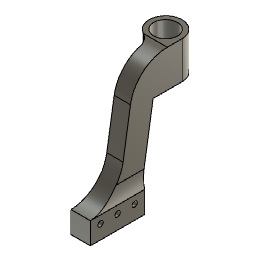
JRCNC0014 v32 (Autodesk Fusion 360 design; units mm, degrees)
Autodesk Fusion 360 part; units mm, degrees
sketch "Sketch1" plane through (0, 0, 0) normal (0, 0, 1) x (1, 0, 0)
  circle A0 centre (0, 0) radius 7.625
  circle A1 centre (0, 0) radius 10.625
  line L0 (0, 0) -> (0, -7.5) construction
  line L1 (10.625, 0) -> (-10.625, 0)
  line L2 (-10.625, 0) -> (-10.625, -15)
  line L3 (-10.625, -15) -> (10.625, -15)
  line L4 (10.625, -15) -> (10.625, 0)
  line L5 (10.625, 0) -> (-10.625, -15) construction
  line L6 (-10.625, 0) -> (10.625, -15) construction
  line L7 (0, 0) -> (0, -15)
  point P0 (0, -7.5)
  dimension "d2" = 3
  dimension "d3" = 15.25
  dimension "d10" = 15
  constraint coincident A0.centre A1.centre
  constraint vertical L0
  constraint horizontal L1
  constraint perpendicular L1 L2
  constraint parallel L1 L3
  constraint parallel L2 L4
  constraint coincident A1 L1.start
  constraint coincident L5 P0
  constraint coincident L6 P0
  constraint coincident P0 L0.end
  constraint midpoint L3 L7.end
  measures "d2" distance of A0 A1
  measures "d3" diameter of A0
  measures "d10" distance of L1.end L2.end
extrude "Extrude1" add sketch "Sketch1" along normal blind 24 contours A0 A1 L1 L7 | A0 A1 L1 | A0 A1 L1 L7 | A1 L3 L4 L7 picked at (1.863551, -9.419618) picked at (-7.385661, 6.132809) picked at (-0.865749, -9.56308) picked at (4.539469, -13.398204)
sketch "Sketch2" plane through (10.625, 0, 0) normal (1, 0, 0) x (0, -1, 0)
  line L0 (15, 0) -> (0, 0)
  line L1 (0, 0) -> (0, -24)
  line L2 (0, -24) -> (15, -24)
  line L3 (15, -24) -> (15, 0)
  line L4 (15, -24) -> (30, -24)
  line L5 (30, -24) -> (41.250246, 46)
  line L6 (41.250246, 46) -> (26.057754, 46)
  line L7 (26.057754, 46) -> (18.656827, -0.049205)
  line L8 (18.656827, -0.049205) -> (15, 0)
  point P0 (33.654, 46)
  dimension "d30" = 30
  dimension "d31" = 70
  dimension "d32" = 33.654
  dimension "d34" = 15
  constraint coincident L2.end L3.start
  constraint perpendicular L3 L4
  constraint perpendicular L3 L6
  constraint parallel L5 L7
  constraint coincident L0.start L3.end
  constraint midpoint L6 P0
  measures "d30" distance of L1 L4.end
  measures "d32" horizontal distance of L0.end P0
  measures "d34" distance of L5 L7
extrude "Extrude2" add sketch "Sketch2" against normal blind 10.5 contours L3 L4 L5 L6 L7 L8 picked at (29.969024, 7.316932)
sketch "Sketch3" plane through (10.625, 0, 0) normal (1, 0, 0) x (0, 1, 0)
  line L0 (0, 24) -> (-30, 24)
  line L1 (-61.057754, -46) -> (-26.057754, -46)
  line L2 (-26.057754, -46) -> (-26.057754, -60)
  line L3 (-26.057754, -60) -> (-61.057754, -60)
  line L4 (-61.057754, -60) -> (-61.057754, -46)
  line L5 (-15, 0) -> (0, 0)
  line L6 (0, 0) -> (0, 24)
  line L7 (-30, 24) -> (-41.250246, -46)
  line L8 (-41.250246, -46) -> (-26.057754, -46)
  line L9 (-26.057754, -46) -> (-18.656827, 0.049205)
  line L10 (-18.656827, 0.049205) -> (-15, 0)
  dimension "d26" = 14
  dimension "d27" = 35
  constraint horizontal L1
  constraint vertical L2
  constraint horizontal L3
  constraint vertical L4
extrude "Extrude3" add sketch "Sketch3" along normal blind 2 and the other way up to surface (10.5 mm away) contours L1 L2 L3 L4 L8 picked at (-42.788585, -55.333333)
sketch "Sketch4" plane through (0.125, 0, 0) normal (-1, 0, 0) x (0, 1, 0)
  line L0 (-61.057754, 51) -> (-26.057754, 51) construction
  line L1 (-30, -24) -> (-15, -24)
  line L2 (-15, -24) -> (-15, 0)
  line L3 (-15, 0) -> (-18.656827, -0.049205)
  line L4 (-18.656827, -0.049205) -> (-26.057754, 46)
  line L5 (-26.057754, 46) -> (-26.057754, 60)
  line L6 (-26.057754, 60) -> (-61.057754, 60)
  line L7 (-61.057754, 60) -> (-61.057754, 46)
  line L8 (-61.057754, 46) -> (-41.250246, 46)
  line L9 (-41.250246, 46) -> (-30, -24)
  point P0 (-54.557754, 51)
  point P1 (-43.557754, 51)
  point P2 (-32.557754, 51)
  dimension "d20" = 11
  dimension "d21" = 11
  dimension "d44" = 5
  constraint horizontal L0
  measures "d44" distance of L0 L8
hole "Hole1" at (0.125, -32.557754, -51) at (0.125, -43.557754, -51) at (0.125, -54.557754, -51) direction (1, 0, 0) diameter 3.4 depth 34 tip angle 180 counterbore diameter 6.5 counterbore depth 7
fillet "Fillet1" radius 9.5 1 edges at (0, -10.625, 12)
fillet "Fillet1" radius 24 3 edges at (5.375, -30, 24) (5.375, -41.250246, -46) (10.625, -33.654, -46)
equation "d32 = 45 mm - 11.346 mm"
